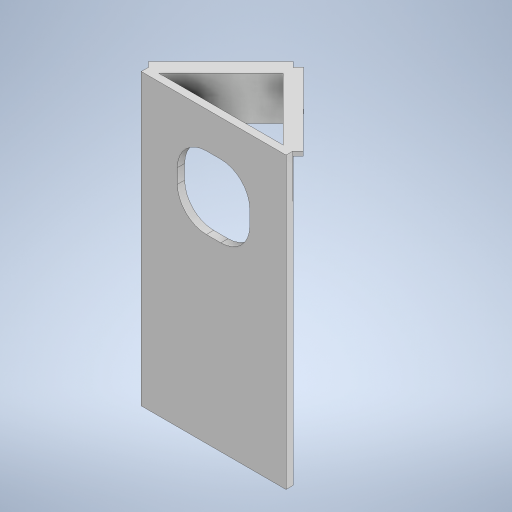
# Autodesk Inventor part: fixation_v09
Saved by Autodesk Inventor 2023 (Build 270158000, 158)
## iProperties
Created: 2021-04-13
Part Number: fixation_v09
Material: Generic
Document SubType Name: Modeling
Designer: KAMPFF-LAB-BEHAVIOR
Density: 1 g/cm^3
Appearance: Default
Author: KAMPFF-LAB-BEHAVIOR
Autodesk Inventor part; units mm, degrees
ref_plane "YZ Plane" through (0, 0, 0) normal (1, 0, 0) x (0, 1, 0)
ref_plane "XZ Plane" through (0, 0, 0) normal (0, 1, 0) x (-1, 0, 0)
ref_plane "XY Plane" through (0, 0, 0) normal (0, 0, 1) x (1, 0, 0)
sketch "Sketch1" plane through (0, 0, 0) normal (0, 0, 1) x (1, 0, 0)
  line L0 (-50, -100) -> (50, -100)
  line L1 (50, -100) -> (50, 100)
  line L2 (50, 100) -> (-50, 100)
  line L3 (-50, 100) -> (-50, -100)
  line L4 (-50, -100) -> (50, 100) construction
  line L5 (50, -100) -> (-50, 100) construction
  point P0 (0, 0)
  dimension "d0" = 100
  dimension "d1" = 200
  constraints: 12 end point, 2 midpoint, 2 parallel, 1 horizontal, 1 perpendicular
  measures "d0" distance of L2.end L1.end
  measures "d1" distance of L1.end L0.end
extrude "Extrusion1" add sketch "Sketch1" along normal blind 5
sketch "Sketch2" plane through (-50, 100, 0) normal (0, 1, 0) x (1, 0, 0)
  line L0 (0, 0) -> (100, 0) projected
  line L1 (0, 0) -> (49.9986, 49.9986)
  line L2 (49.9986, 49.9986) -> (53.5341, 46.463)
  line L3 (53.5341, 46.463) -> (3.5355, -3.5355)
  line L4 (3.5355, -3.5355) -> (0, 0)
  line L5 (0, 0) -> (70.7086, 0) construction
  line L6 (100.108, -0.1109) -> (53.5341, 46.463)
  line L7 (53.5341, 46.463) -> (49.9986, 42.9275)
  line L8 (49.9986, 42.9275) -> (96.5724, -3.6464)
  line L9 (96.5724, -3.6464) -> (100.108, -0.1109)
  point P0 (50, 0)
  point P1 (49.9986, 42.9275)
  dimension "d4" = 45
  dimension "d5" = 5
  dimension "d6" = 5
  constraints: 18 end point, 5 parallel, 2 perpendicular, 1 equal length, 1 horizontal, 1 point on line
  measures "d4" angle of L5 L1
  measures "d5" distance of L1.end L2.end
  measures "d6" distance of L7.end L2.end
extrude "Extrusion2" add sketch "Sketch2" against normal blind 30 contours L1 L2 L3 L0 | L0 L3 L4 | L8 L3 L6 L0 | L0 L6 L9 L8
sketch "Sketch6" plane through (0, 0, 5) normal (0, 0, 1) x (1, 0, 0)
  line L0 (4.9986, 75) -> (-5.0014, 75)
  line L1 (-25.0014, 55) -> (-25.0014, 45)
  line L2 (-5.0014, 25) -> (4.9986, 25)
  line L3 (24.9986, 45) -> (24.9986, 55)
  line L4 (24.9986, 75) -> (-25.0014, 25) construction
  line L5 (-25.0014, 75) -> (24.9986, 25) construction
  arc A0 (4.9986, 25) -> (24.9986, 45) centre (4.9986, 45) ccw
  arc A1 (24.9986, 55) -> (4.9986, 75) centre (4.9986, 55) ccw
  arc A2 (-5.0014, 75) -> (-25.0014, 55) centre (-5.0014, 55) ccw
  arc A3 (-25.0014, 45) -> (-5.0014, 25) centre (-5.0014, 45) ccw
  point P0 (0, 0)
  point P1 (-0.0014, 50)
  dimension "d21" = 50
  dimension "d22" = 50
  dimension "d23" = 20
  constraints: 12 end point, 8 point on circle, 8 point on line, 8 tangent, 4 centre point, 3 equal radius, 2 midpoint, 2 parallel, 1 horizontal, 1 perpendicular
  measures "d21" distance of L5.end L4.end
  measures "d22" distance of L4.end L5.start
  measures "d23" radius of A0
extrude "Extrusion6" cut sketch "Sketch6" against normal blind 5
sketch "Sketch10" plane through (-50, 100, 5) normal (0, 1, 0) x (1, 0, 0)
  line L0 (0, 5) -> (7.0711, 5) projected
  line L1 (49.9986, 54.9986) -> (99.9971, 5) projected
  line L2 (0, 5) -> (49.9986, 54.9986)
  line L3 (49.9986, 54.9986) -> (46.463, 58.5341)
  line L4 (46.463, 58.5341) -> (-3.5355, 8.5355)
  line L5 (-3.5355, 8.5355) -> (0, 5)
  line L6 (100, 4.7812) -> (100, 0) projected
  line L7 (100, 4.7812) -> (49.9986, 54.9986)
  line L8 (49.9986, 54.9986) -> (53.5417, 58.5265)
  line L9 (53.5417, 58.5265) -> (103.5431, 8.3091)
  line L10 (103.5431, 8.3091) -> (100, 4.7812)
  line L11 (92.926, 5) -> (49.9986, 47.9275) projected
  line L12 (100, 0) -> (0, 0) projected
  line L13 (0, 0) -> (100, 0)
  point P0 (50, 5)
  dimension "d33" = 5
  dimension "d34" = 5
  constraints: 18 end point, 4 parallel, 3 perpendicular, 1 horizontal
  measures "d33" distance of L3.end L1.start
  measures "d34" distance of L1.start L8.end
extrude "Extrusion9" add sketch "Sketch10" against normal blind 3
body "Solid1"
